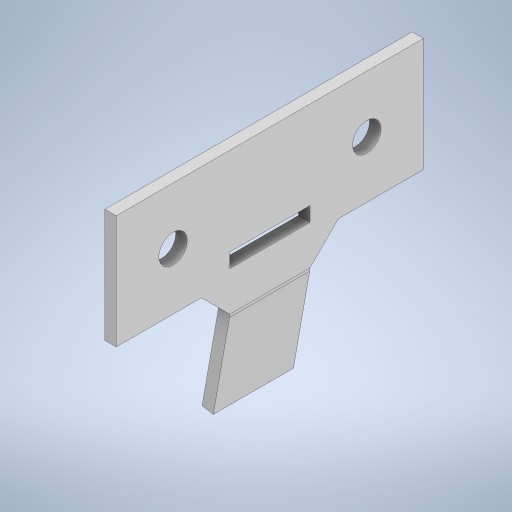
# Autodesk Inventor part: manual_locker_upoper
Saved by Autodesk Inventor 2024 (Build 280153000, 153)
## iProperties
Created: 2025-12-27
Part Number: manual_locker_upoper
Material: Generic
Document SubType Name: Modeling
Designer: schar
Density: 1 g/cm^3
Appearance: Default
Description: Manual Locker Upper Part
Author: schar
Autodesk Inventor part; units mm, degrees
note: some values were not read from the file. Chosen so that the rebuilt part matches the saved one: bend side of "Bend Part1".
ref_plane "YZ Plane" through (0, 0, 0) normal (1, 0, 0) x (0, 1, 0)
ref_plane "XZ Plane" through (0, 0, 0) normal (0, 1, 0) x (-1, 0, 0)
ref_plane "XY Plane" through (0, 0, 0) normal (0, 0, 1) x (1, 0, 0)
sketch "Sketch1" plane through (0, 0, 0) normal (1, 0, 0) x (0, 1, 0)
  line L0 (0, 0) -> (-20, 0)
  line L1 (-20, 0) -> (-20, -54.112)
  line L2 (-20, -54.112) -> (0, -54.112)
  line L3 (0, -54.112) -> (0, 0)
  line L4 (-20, 0) -> (-20, -27.056)
  line L5 (-20, -27.056) -> (-20, -34.112)
  line L6 (-20, -34.112) -> (-42, -34.112)
  line L7 (-42, -34.112) -> (-42, -20)
  line L8 (-42, -20) -> (-20, -20)
  line L9 (-20, -20) -> (-20, -34.112)
  line L10 (-20, -20) -> (-18, -20)
  line L11 (-18, -20) -> (-15.5, -20)
  line L12 (-15.5, -20) -> (-15.5, -34.112)
  line L13 (-15.5, -34.112) -> (-18, -34.112)
  line L14 (-18, -34.112) -> (-18, -20)
  line L15 (-20, -20) -> (-20, -15)
  line L16 (-20, -15) -> (-25, -20)
  line L17 (-20, -34.112) -> (-25, -34.112)
  line L18 (-25, -34.112) -> (-20, -39.112)
  line L19 (-20, -34.112) -> (-20, -39.112)
  dimension "d0" = 20
  dimension "d1" = 54.112
  dimension "d2" = 27.056
  dimension "d3" = 7.056
  dimension "d4" = 22
  dimension "d5" = 14.112
  dimension "d6" = 2
  dimension "d7" = 2.5
  dimension "d8" = 5
  dimension "d9" = 45
  dimension "d10" = 5
  constraints: 40 end point, 6 parallel, 5 point on line, 4 horizontal, 4 perpendicular, 1 midpoint
  measures "d0" distance of L2.end L1.end
  measures "d1" distance of L1.end L0.end
  measures "d2" distance of L0.end L4.end
  measures "d3" distance of L4.end L5.end
  measures "d4" distance of L7.end L8.end
  measures "d5" distance of L6.end L7.end
  measures "d6" distance of L8.end L10.end
  measures "d7" distance of L12.end L13.end
  measures "d8" distance of L8.end L15.end
  measures "d9" angle of L16 L15
  measures "d10" distance of L5.end L17.end
extrude "Extrusion1" add sketch "Sketch1" along normal blind 2
sketch "Sketch2" plane through (2, 0, 0) normal (1, 0, 0) x (0, 0, -1)
  line L0 (20, -25) -> (20, -42) projected
  line L1 (34.112, -42) -> (34.112, -25) projected
  line L2 (20, -25) -> (34.112, -25)
  point P0 (0, 0)
  constraints: 2 end point, 1 horizontal
bend part "Bend Part1" radius 3 angle 10 line through (2, -25, -20) along (0, 0, -1) centre toward (-1, 0, 0) moving side (0, -1, 0) both sides no
sketch "Sketch3" plane through (2, 0, 0) normal (1, 0, 0) x (0, 0, -1)
  line L0 (0, 0) -> (0, -20) projected
  line L1 (0, 0) -> (10, 0)
  line L2 (10, 0) -> (10, -10)
  line L3 (10, -10) -> (0, -10)
  line L4 (0, -10) -> (0, 0)
  line L5 (54.112, 0) -> (0, 0) projected
  line L6 (54.112, 0) -> (44.112, 0)
  line L7 (44.112, 0) -> (44.112, -10)
  line L8 (44.112, -10) -> (54.112, -10)
  line L9 (54.112, -10) -> (54.112, 0)
  circle A0 centre (10, -10) radius 2.5
  circle A1 centre (44.112, -10) radius 2.5
  dimension "d15" = 10
  dimension "d16" = 10
  dimension "d17" = 10
  dimension "d18" = 10
  dimension "d19" = 5
  dimension "d20" = 5
  constraints: 16 end point, 4 parallel, 2 centre point, 2 coincident, 2 horizontal, 2 perpendicular
  measures "d15" distance of L2.end L3.end
  measures "d16" distance of L1.end L2.end
  measures "d17" distance of L8.end L7.end
  measures "d18" distance of L7.end L6.end
  measures "d19" diameter of A0
  measures "d20" diameter of A1
extrude "Extrusion2" cut sketch "Sketch3" against normal blind 2 contours A0 L2 L3 | L3 L2 A0 | A1 L8 L7 | L7 L8 A1
body "Solid1"
